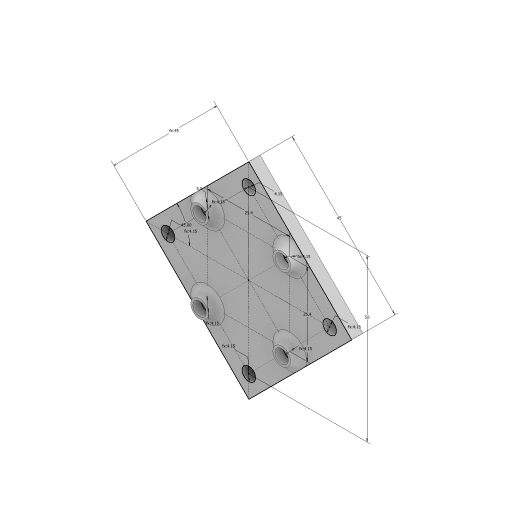
# Autodesk Inventor part: lid_mount_sparkfun_openlog_artemis
Saved by Autodesk Inventor 2023 (Build 270158000, 158)
## iProperties
Created: 2024-08-28
Part Number: lid_mount_sparkfun_openlog_artemis
Material: Generic
Document SubType Name: Modeling
Designer: Thomas
Density: 1 g/cm^3
Appearance: Default
Author: Thomas
Autodesk Inventor part; units mm, degrees
ref_plane "YZ Plane" through (0, 0, 0) normal (1, 0, 0) x (0, 1, 0)
ref_plane "XZ Plane" through (0, 0, 0) normal (0, 1, 0) x (-1, 0, 0)
ref_plane "XY Plane" through (0, 0, 0) normal (0, 0, 1) x (1, 0, 0)
sketch "Sketch1" plane through (0, 0, 0) normal (0, 0, 1) x (1, 0, 0)
  line L0 (-25, 0) -> (0, 25) construction
  line L1 (0, 25) -> (25, 0) construction
  line L2 (25, 0) -> (0, -25) construction
  line L3 (0, -25) -> (-25, 0) construction
  line L4 (-25, 0) -> (25, 0) construction
  line L5 (0, 25) -> (0, -25) construction
  circle A0 centre (0, 25) radius 2.075
  circle A1 centre (25, 0) radius 2.075
  circle A2 centre (0, -25) radius 2.075
  circle A3 centre (-25, 0) radius 2.075
  line L6 (-12.7, -12.7) -> (12.7, -12.7) construction
  line L7 (12.7, -12.7) -> (12.7, 12.7) construction
  line L8 (12.7, 12.7) -> (-12.7, 12.7) construction
  line L9 (-12.7, 12.7) -> (-12.7, -12.7) construction
  line L10 (-12.7, -12.7) -> (12.7, 12.7) construction
  line L11 (12.7, -12.7) -> (-12.7, 12.7) construction
  circle A4 centre (-12.7, 12.7) radius 2.075
  circle A5 centre (12.7, 12.7) radius 2.075
  circle A6 centre (12.7, -12.7) radius 2.075
  circle A7 centre (-12.7, -12.7) radius 2.075
  circle A8 centre (-12.7, 12.7) radius 2.75
  line L12 (-31.8198, 0) -> (0, 31.8198)
  line L13 (0, 31.8198) -> (31.8198, 0)
  line L14 (31.8198, 0) -> (0, -31.8198)
  line L15 (0, -31.8198) -> (-31.8198, 0)
  line L16 (-31.8198, 0) -> (13.1802, 0) construction
  line L17 (0, 31.8198) -> (0, -31.8198) construction
  point P0 (0, 0)
  point P1 (0, 0)
  point P2 (0, 0)
  dimension "d0" = 50
  dimension "d1" = 4.15
  dimension "d2" = 4.15
  dimension "d3" = 4.15
  dimension "d4" = 4.15
  dimension "d5" = 25.4
  dimension "d6" = 25.4
  dimension "d7" = 4.15
  dimension "d8" = 4.15
  dimension "d9" = 4.15
  dimension "d10" = 4.15
  dimension "d11" = 5.5
  dimension "d12" = 45
  dimension "d13" = 45
  dimension "d18" = 45
  constraints: 36 end point, 13 coincident, 9 centre point, 6 parallel, 5 midpoint, 3 horizontal, 3 perpendicular, 1 equal length, 1 point on line, 1 vertical
  measures "d0" distance of L0.end L2.end
  measures "d1" diameter of A0
  measures "d2" diameter of A1
  measures "d3" diameter of A2
  measures "d4" diameter of A3
  measures "d5" distance of L8.end L7.end
  measures "d6" distance of L7.end L6.end
  measures "d7" diameter of A4
  measures "d8" diameter of A5
  measures "d9" diameter of A6
  measures "d10" diameter of A7
  measures "d11" diameter of A8
  measures "d12" angle of L16 L12
  measures "d13" distance of L12.end L13.end
  measures "d18" distance of L12.start L12.end
extrude "Extrusion1" add sketch "Sketch1" against normal blind 3.5 contours A8 | L12 L13 L14 L15
extrude "Extrusion2" add sketch "Sketch1" along normal blind 2.5 contours A8
pattern_sketch "Sketch Driven Pattern1" of "Extrusion2" from (-12.7, 12.7, 0) copies at (12.7, 12.7, 0) at (12.7, -12.7, 0) at (-12.7, -12.7, 0)
fillet "Fillet1" radius 2.5 4 edges at (-15.45, 12.7, 0) (9.95, 12.7, 0) (9.95, -12.7, 0) (-15.45, -12.7, 0)
equation "\"d2\" = d1"
equation "\"d3\" = d1"
equation "\"d4\" = d1"
equation "\"d7\" = d1"
equation "\"d8\" = d1"
equation "\"d9\" = d1"
equation "\"d10\" = d1"
equation "\"d18\" = d13"
body "Solid1"
